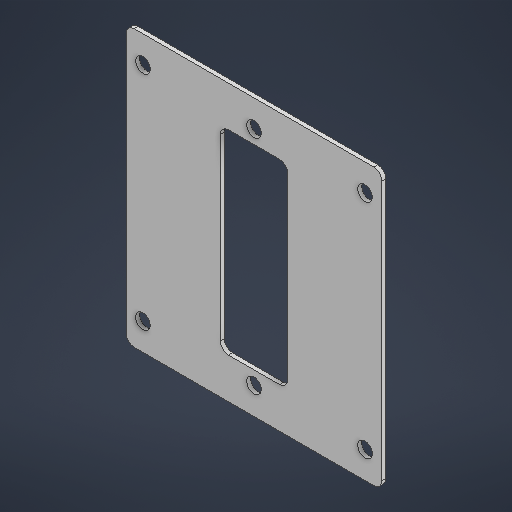
# Autodesk Inventor part: DMF 2.1 01 42 Gear way 2
Saved by Autodesk Inventor 2026.2 (Build 302298010, 298A)
## iProperties
Created: 2024-04-30
Part Number: DMF 2.1 01 42 Gear way 2
Material: Generic
Document SubType Name: Sheet Metal
Designer: admin
Stock Number: Барабан_Сектор_Усилителя
Density: 1 g/cm^3
Sheet Metal Rule: Default
Sheet Metal Width: 190,000 mm
Sheet Metal Length: 205,000 mm
Sheet Metal Area: 38950,000 mm^2
Appearance: Default
Flat Pattern Width: 19 cm
Flat Pattern Length: 20.5 cm
Flat Pattern Area: 389.5 cm^2
d68: 145,000 mm
d69: 50,000 mm
Author: pokla
Autodesk Inventor part; units mm, degrees
ref_plane "YZ Plane" through (0, 0, 0) normal (1, 0, 0) x (0, 1, 0)
ref_plane "XZ Plane" through (0, 0, 0) normal (0, 1, 0) x (-1, 0, 0)
ref_plane "XY Plane" through (0, 0, 0) normal (0, 0, 1) x (1, 0, 0)
sketch "Sketch1" plane through (0, 0, 0) normal (0, 0, 1) x (1, 0, 0)
  line L0 (-95, 205) -> (95, 205)
  line L1 (95, 205) -> (95, 0)
  line L2 (95, 0) -> (-95, 0)
  line L3 (-95, 0) -> (-95, 205)
  point P0 (0, 0)
  point P1 (0, 0)
  point P2 (0, 0)
  point P3 (0, 0)
  point P4 (0, 0)
  dimension "d27" = 190
  dimension "d29" = 205
  measures "d27" distance of L1.end L2.end
  measures "d29" distance between parallel lines of L2 L0
extrude "Plate1" add sketch "Sketch1" along normal mid plane 3
sketch "Sketch4" plane through (0, 0, -1.5) normal (0, 0, -1) x (-1, 0, 0)
  line L0 (95, 205) -> (-95, 205) construction
  line L1 (-95, 205) -> (-95, 0) construction
  line L2 (-95, 0) -> (95, 0) construction
  line L3 (95, 0) -> (95, 205) construction
  line L4 (-25, 175) -> (25, 175)
  line L5 (25, 175) -> (25, 30)
  line L6 (25, 30) -> (-25, 30)
  line L7 (-25, 30) -> (-25, 175)
  line L8 (-25, 175) -> (25, 30) construction
  line L9 (25, 175) -> (-25, 30) construction
  circle A0 centre (0, 185) radius 5.5
  circle A1 centre (0, 20) radius 5.5
  circle A2 centre (82.5, 20) radius 5.5
  circle A3 centre (82.5, 185) radius 5.5
  circle A4 centre (-82.5, 185) radius 5.5
  circle A5 centre (-82.5, 20) radius 5.5
  line L10 (0, 175) -> (0, 30) construction
  line L11 (-25, 102.5) -> (25, 102.5) construction
  point P0 (0, 0)
  point P1 (0, 102.5)
  point P2 (95, 102.5)
  point P3 (0, 205)
  point P4 (0, 102.5)
  dimension "d51" = 50
  dimension "d52" = 145
  dimension "d53" = 11
  dimension "d54" = 165
  dimension "d70" = 165
  dimension "d71" = 165
  constraints: 18 end point, 9 midpoint, 6 centre point, 2 equal radius, 2 parallel, 2 vertical alignment, 1 horizontal, 1 horizontal alignment, 1 perpendicular, 4 other
  measures "d51" distance of L4.start L4.end
  measures "d52" distance of L6.end L4.start
  measures "d53" diameter of A0
  measures "d54" distance of A1.centre A0.centre
  measures "d70" distance of A4.centre A3.centre
  measures "d71" distance of A4.centre A5.centre
extrude "Cut1" cut sketch "Sketch4" against normal blind 3
fillet "Corner Round1" radius 6 8 edges at (95, 205, 0) (95, 0, 0) (-95, 0, 0) (-95, 205, 0) (25, 30, 0) (-25, 30, 0) (25, 175, 0) (-25, 175, 0)
equation "\"d71\" = d70"
equation "\"d57\" = Thickness"
equation "\"d15\" = Thickness"
equation "\"BendRadius\" = Thickness"
equation "\"BendReliefWidth\" = Thickness"
equation "\"BendReliefDepth\" = 0.5 * Thickness"
equation "\"CornerReliefSize\" = 4 * Thickness"
equation "\"MinimumRemnant\" = 2 * Thickness"
equation "\"TransitionRadius\" = BendRadius"
equation "\"JacobiRadiusSize\" = BendRadius"
equation "\"GapSize\" = Thickness"
equation "\"d68\" = 145"
equation "\"Thickness\" = 3"
body "Solid1"
